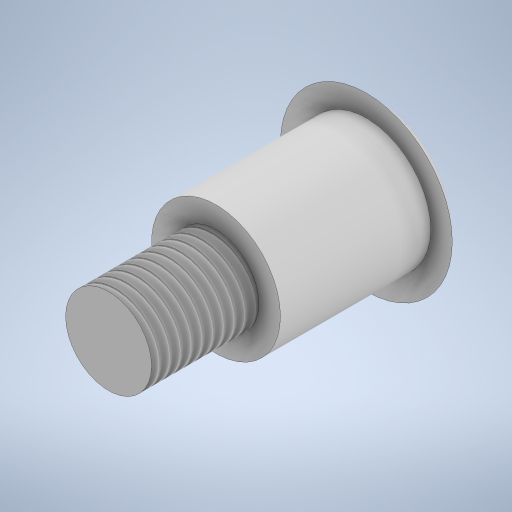
# Autodesk Inventor part: m2mit025
Saved by Autodesk Inventor 2023 (Build 270158000, 158)
## iProperties
Created: 2022-05-26
Part Number: m2mit025
Material: Generisch
Document SubType Name: Modeling
Designer: Tim Stechel
Density: 1 g/cm^3
Appearance: Vorgabe
Author: Tim Stechel
Autodesk Inventor part; units mm, degrees
ref_plane "YZ Plane" through (0, 0, 0) normal (1, 0, 0) x (0, 1, 0)
ref_plane "XZ Plane" through (0, 0, 0) normal (0, 1, 0) x (-1, 0, 0)
ref_plane "XY Plane" through (0, 0, 0) normal (0, 0, 1) x (1, 0, 0)
sketch "Skizze1" plane through (0, 0, 0) normal (0, 0, 1) x (1, 0, 0)
  circle A0 centre (0, 0) radius 1.5
  dimension "d0" = 3
  constraints: 1 centre point, 1 coincident
  measures "d0" diameter of A0
extrude "Extrusion1" add sketch "Skizze1" along normal blind 3.5
sketch "Skizze2" plane through (0, 0, 3.5) normal (0, 0, 1) x (1, 0, 0)
  circle A0 centre (0, 0) radius 1
  dimension "d3" = 2
  constraints: 1 centre point, 1 coincident
  measures "d3" diameter of A0
extrude "Extrusion2" add sketch "Skizze2" along normal blind 2.5
sketch "Skizze3" plane through (0, 0, 0) normal (0, 1, 0) x (-1, 0, 0)
  line L0 (0, 0) -> (2, 0)
  line L1 (1.5, 0) -> (-1.5, 0) projected
  arc A0 (-2, 0) -> (2, 0) centre (0, 1.8875) ccw
  line L2 (0, 0) -> (0, -0.8625)
  dimension "d6" = 2
  dimension "d7" = 4
  dimension "d8" = 2.75
  constraints: 4 end point, 3 point on circle, 1 centre point, 1 collinear, 1 point on line
  measures "d6" distance of L0.start L0.end
  measures "d7" distance of L0.end A0.start
  measures "d8" radius of A0
revolve "Umdrehung1" add sketch "Skizze3" angle 360 about axis through (0, 0, 0) along (0, 0, -1)
thread "Gewinde1" size "M2x0.25" class "6g" standard "ANSI Metric M Profile" length 10
